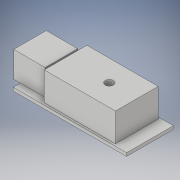
# Autodesk Inventor part: POE splitter
Saved by Autodesk Inventor 2018 (Build 220112000, 112)
## iProperties
Created: 2019-09-13
Part Number: POE splitter
Material: Generic
Document SubType Name: Modeling
Designer: Jacob
Density: 1 g/cm^3
Appearance: Default
Author: Jacob
Autodesk Inventor part; units mm, degrees
ref_plane "YZ Plane" through (0, 0, 0) normal (1, 0, 0) x (0, 1, 0)
ref_plane "XZ Plane" through (0, 0, 0) normal (0, 1, 0) x (-1, 0, 0)
ref_plane "XY Plane" through (0, 0, 0) normal (0, 0, 1) x (1, 0, 0)
sketch "Sketch1" plane through (0, 0, 0) normal (0, 1, 0) x (-1, 0, 0)
  line L0 (27.875, 11.5) -> (-27.875, 11.5)
  line L1 (-27.875, 11.5) -> (-27.875, -11.5)
  line L2 (-27.875, -11.5) -> (27.875, -11.5)
  line L3 (27.875, -11.5) -> (27.875, 11.5)
  line L4 (27.875, 11.5) -> (-27.875, -11.5) construction
  line L5 (-27.875, 11.5) -> (27.875, -11.5) construction
  point P0 (0, 0)
  dimension "d0" = 23
  dimension "d1" = 55.75
  constraints: 12 end point, 2 midpoint, 2 parallel, 1 horizontal, 1 perpendicular
  measures "d0" distance of L2.end L0.start
  measures "d1" distance of L1.end L2.end
extrude "Extrusion1" add sketch "Sketch1" along normal blind 1.6
sketch "Sketch2" plane through (0, 1.6, 0) normal (0, 1, 0) x (1, 0, 0)
  line L0 (-27.875, 11.5) -> (-27.875, -11.5) projected
  line L1 (-27.875, 0) -> (27.875, 0) construction
  line L2 (27.875, -11.5) -> (27.875, 11.5) projected
  line L3 (27.875, 11.5) -> (-27.875, 11.5) projected
  line L4 (0, 11.5) -> (0, -11.5) construction
  line L5 (-27.875, -11.5) -> (27.875, -11.5) projected
  line L6 (-31.125, -8) -> (-15.625, -8)
  line L7 (-15.625, -8) -> (-15.625, 8)
  line L8 (-15.625, 8) -> (-31.125, 8)
  line L9 (-31.125, 8) -> (-31.125, -8)
  line L10 (-31.125, -8) -> (-15.625, 8) construction
  line L11 (-15.625, -8) -> (-31.125, 8) construction
  line L12 (-31.125, 0) -> (-31.125, 11.7412) construction
  point P0 (0, 0)
  point P1 (-23.375, 0)
  dimension "d5" = 15.5
  dimension "d6" = 16
  dimension "d7" = 3.25
  dimension "d9" = 0
  constraints: 18 end point, 6 midpoint, 2 parallel, 1 horizontal, 1 perpendicular, 1 point on line, 1 vertical
  measures "d5" distance of L7.end L8.end
  measures "d6" distance of L6.end L7.end
  measures "d7" distance between parallel lines of L0 L12
  measures "d9" distance between parallel lines of L12 L9
extrude "Extrusion2" add sketch "Sketch2" along normal blind 12.75 contours L8 L7 L6 L0 | L0 L6 L9 L8
sketch "Sketch3" plane through (0, 1.6, 0) normal (0, 1, 0) x (1, 0, 0)
  line L0 (27.875, -11.5) -> (27.875, 11.5) projected
  line L1 (27.875, 0) -> (0, 0) construction
  line L2 (-13.625, -10.5) -> (21.375, -10.5)
  line L3 (21.375, -10.5) -> (21.375, 10.5)
  line L4 (21.375, 10.5) -> (-13.625, 10.5)
  line L5 (-13.625, 10.5) -> (-13.625, -10.5)
  line L6 (-13.625, -10.5) -> (21.375, 10.5) construction
  line L7 (21.375, -10.5) -> (-13.625, 10.5) construction
  point P0 (3.875, 0)
  dimension "d12" = 6.5
  dimension "d13" = 21
  dimension "d14" = 35
  constraints: 14 end point, 3 midpoint, 2 horizontal, 2 parallel, 1 perpendicular, 1 point on line
  measures "d12" distance between parallel lines of L0 L3
  measures "d13" distance of L2.end L3.end
  measures "d14" distance of L3.end L4.end
extrude "Extrusion3" add sketch "Sketch3" along normal blind 14
sketch "Sketch4" plane through (0, 0, 0) normal (0, -1, 0) x (1, 0, 0)
  line L0 (27.7099, 0) -> (-27.875, 0) construction
  line L1 (-27.875, -11.5) -> (-27.875, 11.5) projected
  circle A0 centre (7.875, 0) radius 2
  line L2 (27.875, 11.5) -> (27.875, -11.5) projected
  point P0 (0, 0)
  dimension "d17" = 20
  dimension "d18" = 4
  constraints: 2 end point, 1 centre point, 1 midpoint, 1 point on line
  measures "d17" distance from line of L2 A0.centre
  measures "d18" diameter of A0
extrude "Extrusion4" cut sketch "Sketch4" against normal blind 25.4
body "Solid1"
